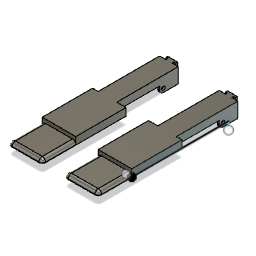
WhiteKeyCLRNew (Autodesk Fusion 360 design; units mm, degrees)
Autodesk Fusion 360 part; units mm, degrees
sketch "Sketch1" plane through (0, 0, 0) normal (0, 1, 0) x (1, 0, 0)
  line L0 (43.1546, -52.768) -> (20.2946, -52.768)
  line L1 (43.1546, -18.478) -> (43.1546, -52.768)
  line L2 (20.2946, -52.768) -> (20.2946, -50.8)
  line L3 (38.1, 23.432) -> (22.86, 23.432)
  line L4 (20.2946, -18.478) -> (20.2946, -52.768)
  line L5 (20.2946, -18.478) -> (22.86, -18.478)
  line L6 (22.86, -18.478) -> (22.86, 23.432)
  line L7 (38.1, 23.432) -> (38.1, -18.478)
  line L8 (38.1, -18.478) -> (43.1546, -18.478)
  dimension "d3" = 22.86
  dimension "d91" = 15.24
  dimension "d119" = 76.2
  dimension "d157" = 5.0546
  constraint horizontal L0
  constraint perpendicular L0 L2
  constraint perpendicular L1 L3
  constraint perpendicular L0 L4
  constraint perpendicular L4 L5
  constraint perpendicular L3 L6
  constraint perpendicular L3 L7
  constraint perpendicular L1 L8
  measures "d3" distance of L0.start L0.end
  measures "d91" distance of L3.end L3.start
  measures "d119" distance of L0 L3
  measures "d157" distance of L7.end L1.start
extrude "Extrude1" add sketch "Sketch1" along normal blind 5.08 makes body 1
sketch "Sketch18" plane through (0, 0, 0) normal (0, -1, 0) x (1, 0, 0)
  line L0 (22.86, -23.432) -> (38.1, -23.432)
  line L1 (38.1, -23.432) -> (38.1, 18.478)
  line L2 (38.1, 18.478) -> (43.1546, 18.478)
  line L3 (43.1546, 18.478) -> (43.1546, 52.768)
  line L4 (43.1546, 52.768) -> (20.2946, 52.768)
  line L5 (20.2946, 52.768) -> (20.2946, 18.478)
  line L6 (20.2946, 18.478) -> (22.86, 18.478)
  line L7 (22.86, 18.478) -> (22.86, -23.432)
  line L8 (35.56, -20.892) -> (35.56, 21.018)
  line L9 (35.56, 21.018) -> (40.6146, 21.018)
  line L10 (40.6146, 21.018) -> (40.6146, 50.228)
  line L11 (40.6146, 50.228) -> (22.8346, 50.228)
  line L12 (22.8346, 50.228) -> (22.8346, 21.018)
  line L13 (22.8346, 21.018) -> (25.4, 21.018)
  line L14 (35.56, -20.892) -> (25.4, -20.892)
  line L15 (25.4, -20.892) -> (25.4, 21.018)
  dimension "d130" = 2.54
  dimension "d131" = 2.54
  dimension "d132" = 2.54
  dimension "d133" = 2.54
  dimension "d134" = 2.54
  dimension "d135" = 2.54
  dimension "d136" = 2.54
  dimension "d137" = 2.54
  constraint perpendicular L0 L8
  constraint perpendicular L8 L9
  constraint perpendicular L9 L10
  constraint perpendicular L10 L11
  constraint perpendicular L11 L12
  constraint perpendicular L12 L13
  constraint perpendicular L8 L14
  constraint perpendicular L14 L15
  measures "d130" distance of L1 L8
  measures "d131" distance of L7 L15
  measures "d132" distance of L0 L14
  measures "d133" distance of L5 L12
  measures "d134" distance of L6 L13
  measures "d135" distance of L2 L9
  measures "d136" distance of L3 L10
  measures "d137" distance of L4 L11
extrude "Extrude20" cut sketch "Sketch18" against normal blind 3.81 contours L8 L9 L10 L11 L12 L13 L14 L15 bodies 1
sketch "Sketch19" plane through (0, 0, 0) normal (0, -1, 0) x (1, 0, 0)
  line L0 (40.6146, 21.018) -> (35.56, 21.018)
  line L1 (35.56, 21.018) -> (35.56, -20.892)
  line L2 (35.56, -20.892) -> (25.4, -20.892)
  line L3 (25.4, -20.892) -> (25.4, 21.018)
  line L4 (25.4, 21.018) -> (22.8346, 21.018)
  line L5 (22.8346, 21.018) -> (22.8346, 50.228)
  line L6 (22.8346, 50.228) -> (40.6146, 50.228)
  line L7 (40.6146, 50.228) -> (40.6146, 21.018)
  line L8 (22.86, -23.432) -> (38.1, -23.432)
  line L9 (38.1, -23.432) -> (38.1, 18.478)
  line L10 (38.1, 18.478) -> (43.1546, 18.478)
  line L11 (43.1546, 18.478) -> (43.1546, 52.768)
  line L12 (43.1546, 52.768) -> (20.2946, 52.768)
  line L13 (20.2946, 52.768) -> (20.2946, 18.478)
  line L14 (20.2946, 18.478) -> (22.86, 18.478)
  line L15 (22.86, 18.478) -> (22.86, -23.432)
  line L16 (35.56, -10.732) -> (38.1, -10.732)
  line L17 (38.1, -10.732) -> (38.1, -23.432)
  line L18 (38.1, -23.432) -> (35.56, -23.432)
  line L19 (35.56, -23.432) -> (35.56, -10.732)
  line L20 (22.86, -10.732) -> (26.162, -10.732)
  line L21 (26.162, -10.732) -> (26.162, -23.432)
  line L22 (26.162, -23.432) -> (22.86, -23.432)
  line L23 (22.86, -23.432) -> (22.86, -10.732)
  line L24 (25.4, -20.892) -> (35.56, -20.892)
  line L25 (35.56, -20.892) -> (35.56, -23.432)
  line L26 (35.56, -23.432) -> (25.4, -23.432)
  line L27 (25.4, -23.432) -> (25.4, -20.892)
  dimension "d149" = 12.7
  dimension "d150" = 12.7
  constraint horizontal L16
  constraint vertical L17
  constraint horizontal L18
  constraint vertical L19
  constraint coincident L8.end L9.start
  constraint coincident L1 L16.start
  constraint horizontal L20
  constraint vertical L21
  constraint horizontal L22
  constraint vertical L23
  constraint coincident L8 L21.end
  constraint coincident L15 L20.start
  constraint horizontal L24
  constraint vertical L25
  constraint horizontal L26
  constraint vertical L27
  constraint coincident L2.end L3.start
  measures "d149" distance of L16.start L18.end
  measures "d150" distance of L20.end L21.end
extrude "Extrude21" add sketch "Sketch19" along normal blind 5.08 contours L1 L8 L9 L16 L17 L18 L19 L25 | L3 L8 L15 L20 L22 L23 L27 bodies 1
fillet "Fillet7" radius 2.54 2 edges at (36.83, -5.08, -10.732) (24.13, -5.08, -10.732) on bodies 1
sketch "Sketch20" plane through (0, 0, 0) normal (0, -1, 0) x (1, 0, 0)
  line L0 (38.1, -10.732) -> (38.1, 18.478)
  line L1 (38.1, 18.478) -> (43.1546, 18.478)
  line L2 (43.1546, 18.478) -> (43.1546, 52.768)
  line L3 (43.1546, 52.768) -> (20.2946, 52.768)
  line L4 (20.2946, 52.768) -> (20.2946, 18.478)
  line L5 (20.2946, 18.478) -> (22.86, 18.478)
  line L6 (22.86, 18.478) -> (22.86, -10.732)
  line L7 (25.4, -10.732) -> (25.4, 21.018)
  line L8 (25.4, 21.018) -> (22.8346, 21.018)
  line L9 (22.8346, 21.018) -> (22.8346, 50.228)
  line L10 (22.8346, 50.228) -> (40.6146, 50.228)
  line L11 (40.6146, 50.228) -> (40.6146, 21.018)
  line L12 (40.6146, 21.018) -> (35.56, 21.018)
  line L13 (35.56, 21.018) -> (35.56, -10.732)
  line L14 (22.86, 18.478) -> (25.4, 18.478)
  line L15 (25.4, 18.478) -> (25.4, 12.3012)
  line L16 (25.4, 12.3012) -> (22.86, 12.3012)
  line L17 (22.86, 12.3012) -> (22.86, 18.478)
  line L18 (38.1, 18.478) -> (35.56, 18.478)
  line L19 (35.56, 18.478) -> (35.56, 12.3012)
  line L20 (35.56, 12.3012) -> (38.1, 12.3012)
  line L21 (38.1, 12.3012) -> (38.1, 18.478)
  line L22 (22.86, -10.732) -> (25.4, -10.732)
  line L23 (35.56, -10.732) -> (38.1, -10.732)
  constraint horizontal L14
  constraint vertical L15
  constraint horizontal L16
  constraint vertical L17
  constraint coincident L7 L15.end
  constraint coincident L5.end L6.start
  constraint horizontal L18
  constraint vertical L19
  constraint horizontal L20
  constraint vertical L21
  constraint coincident L13 L19.end
  constraint coincident L0.end L1.start
sketch "Sketch22" plane through (0, 0, -23.432) normal (0, 0, -1) x (-1, 0, 0)
  line L0 (-22.86, -5.08) -> (-22.86, 5.08)
  line L1 (-22.86, 5.08) -> (-38.1, 5.08)
  line L2 (-38.1, 5.08) -> (-38.1, -5.08)
  line L3 (-25.4, -5.08) -> (-22.86, -5.08)
  line L4 (-38.1, 5.08) -> (-22.86, 5.08)
  line L5 (-22.86, 5.08) -> (-22.86, 0)
  line L6 (-22.86, 0) -> (-38.1, 0)
  line L7 (-38.1, 0) -> (-38.1, 5.08)
  line L8 (-35.56, 0) -> (-25.4, 0)
  line L9 (-25.4, 0) -> (-25.4, -5.08)
  line L10 (-38.1, -5.08) -> (-35.56, -5.08)
  line L11 (-35.56, -5.08) -> (-35.56, 0)
  constraint horizontal L4
  constraint vertical L5
  constraint horizontal L6
  constraint vertical L7
  constraint midpoint L0 L5.end
  constraint coincident L1.end L2.start
extrude "Extrude24" add sketch "Sketch22" along normal blind 2.54 contours L0 L1 L2 L4 L5 L6 L7 L8 bodies 1
sketch "Sketch23" plane through (38.1, 0, 0) normal (1, 0, 0) x (0, 0, -1)
  arc A0 (10.732, -2.54) -> (13.272, -5.08) centre (13.272, -2.54) ccw
  line L0 (13.272, -5.08) -> (23.432, -5.08)
  line L1 (23.432, -5.08) -> (23.432, 0)
  line L2 (23.432, 0) -> (25.972, 0)
  line L3 (25.972, 0) -> (25.972, 5.08)
  line L4 (25.972, 5.08) -> (-18.478, 5.08)
  line L5 (-18.478, 5.08) -> (-18.478, 0)
  line L6 (-18.478, 0) -> (10.732, 0)
  line L7 (23.432, 0) -> (24.702, 0)
  line L8 (24.702, 0) -> (24.702, 3.81)
  line L9 (24.702, 3.81) -> (23.432, 3.81)
  line L10 (23.432, 3.81) -> (23.432, 0)
  line L11 (10.732, 0) -> (10.732, -2.54)
  dimension "d160" = 1.27
  constraint horizontal L7
  constraint vertical L8
  constraint horizontal L9
  constraint vertical L10
  constraint coincident L1.end L2.start
  measures "d160" distance of L1.end L7.end
extrude "Extrude25" cut sketch "Sketch23" against normal blind 1.27 contours L2 L7 L8 L9 L10 bodies 1
sketch "Sketch24" plane through (22.86, 0, 0) normal (-1, 0, 0) x (0, 0, 1)
  arc A0 (-13.272, -5.08) -> (-10.732, -2.54) centre (-13.272, -2.54) ccw
  line L0 (-10.732, 0) -> (18.478, 0)
  line L1 (18.478, 0) -> (18.478, 5.08)
  line L2 (18.478, 5.08) -> (-25.972, 5.08)
  line L3 (-25.972, 5.08) -> (-25.972, 0)
  line L4 (-25.972, 0) -> (-23.432, 0)
  line L5 (-23.432, 0) -> (-23.432, -5.08)
  line L6 (-23.432, -5.08) -> (-13.272, -5.08)
  line L7 (-23.432, 0) -> (-24.702, 0)
  line L8 (-24.702, 0) -> (-24.702, 3.81)
  line L9 (-24.702, 3.81) -> (-23.432, 3.81)
  line L10 (-23.432, 3.81) -> (-23.432, 0)
  line L11 (-10.732, -2.54) -> (-10.732, 0)
  dimension "d163" = 1.27
  constraint horizontal L7
  constraint vertical L8
  constraint horizontal L9
  constraint vertical L10
  constraint coincident L4.end L5.start
  measures "d163" distance of L4.end L7.end
extrude "Extrude26" cut sketch "Sketch24" against normal blind 1.27 contours L4 L7 L8 L9 L10 bodies 1
move_body "Move1" bodies 1 to x (1, 0, 0) y (0, 1, 0) z (0, 0, 1) at (-50.8, 0, 0)
sketch "Sketch25" plane through (0, 0, 52.768) normal (0, 0, 1) x (1, 0, 0)
  line L0 (-30.5054, 0) -> (-7.6454, 0)
  line L1 (-7.6454, 0) -> (-7.6454, 5.08)
  line L2 (-7.6454, 5.08) -> (-30.5054, 5.08)
  line L3 (-30.5054, 5.08) -> (-30.5054, 0)
  line L4 (-30.5054, 2.54) -> (-7.6454, 2.54)
  constraint midpoint L3 L4.start
  constraint midpoint L1 L4.end
extrude "Extrude27" add sketch "Sketch25" along normal blind 22.86 contours L0 L1 L3 L4 bodies 1
fillet "Fillet8" radius 2.286 5 edges at (-7.6454, 1.27, 75.628) (-7.6454, 2.54, 64.198) (-19.0754, 2.54, 75.628) (-30.5054, 2.54, 64.198) (-30.5054, 1.27, 75.628) on bodies 1
sketch "Sketch26" plane through (-12.7, 0, 0) normal (1, 0, 0) x (0, 0, -1)
  line L0 (23.432, -5.08) -> (23.432, 3.81)
  line L1 (25.972, 5.08) -> (-18.478, 5.08)
  line L2 (-18.478, 5.08) -> (-18.478, 0)
  line L3 (24.702, 0) -> (25.972, 0)
  line L4 (10.732, 0) -> (10.732, -2.54)
  arc A0 (10.732, -2.54) -> (13.272, -5.08) centre (13.272, -2.54) ccw
  line L5 (13.272, -5.08) -> (23.432, -5.08)
  circle A1 centre (13.272, -2.54) radius 1.27
  line L6 (24.702, 3.81) -> (24.702, 0)
  line L7 (25.972, 0) -> (25.972, 5.08)
  line L8 (23.432, 3.81) -> (24.702, 3.81)
  line L9 (-18.478, 0) -> (10.732, 0)
  dimension "d174" = 2.54
  constraint concentric A0 A1
  measures "d174" diameter of A1
extrude "Extrude28" cut sketch "Sketch26" against normal blind 25.4 contours A1 bodies 1
mirror "Mirror4" about plane through (0, 0, 0) normal (1, 0, 0) of bodies 1 makes body 2
extrude "Extrude29" cut 1 faces at (26.67, 1.27, -23.8553) along direction (-1, 0, 0) blind 1.27 on bodies 2 bodies 2
extrude "Extrude30" cut 1 faces at (27.94, -1.2069, -20.4639) along direction (-1, 0, 0) blind 1.27 on bodies 2 bodies 2
extrude "Extrude31" cut 1 faces at (13.97, 1.27, -23.8553) along direction (1, 0, 0) blind 1.27 on bodies 2 bodies 2
extrude "Extrude32" cut 1 faces at (12.7, -1.2069, -20.4639) along direction (1, 0, 0) blind 1.27 on bodies 2 bodies 2
extrude "Extrude33" cut 1 faces at (-13.97, 1.27, -23.8553) along direction (-1, 0, 0) blind 1.27 on bodies 1 bodies 1
extrude "Extrude34" cut 1 faces at (-12.7, -1.2069, -20.4639) along direction (-1, 0, 0) blind 1.27 on bodies 1 bodies 1
extrude "Extrude35" cut 1 faces at (-26.67, 1.27, -23.8553) along direction (1, 0, 0) blind 1.27 on bodies 1 bodies 1
extrude "Extrude36" cut 1 faces at (-27.94, -1.2069, -20.4639) along direction (1, 0, 0) blind 1.27 on bodies 1 bodies 1
extrude "Extrude37" cut 1 faces at (26.2467, 3.81, -24.2787) along direction (0, 1, 0) blind 3.302 on bodies 2 bodies 2
extrude "Extrude38" cut 1 faces at (14.3933, 3.81, -24.2787) along direction (0, 1, 0) blind 3.556 on bodies 2 bodies 2
extrude "Extrude39" cut 1 faces at (-26.2467, 3.81, -24.2787) along direction (0, 1, 0) blind 1.27 on bodies 1 bodies 1
extrude "Extrude40" cut 1 faces at (-14.3933, 3.81, -24.2787) along direction (0, 1, 0) blind 2.794 on bodies 1 bodies 1
sketch "Sketch28" plane through (0, 5.08, 0) normal (0, 1, 0) x (-1, 0, 0)
  line L0 (-15.24, -23.432) -> (-13.97, -23.432)
  line L1 (-13.97, -23.432) -> (-13.97, 18.478)
  line L2 (-13.97, 18.478) -> (-7.6454, 18.478)
  line L3 (-7.6454, 18.478) -> (-7.6454, 52.768)
  line L4 (-7.6454, 52.768) -> (-30.5054, 52.768)
  line L5 (-30.5054, 52.768) -> (-30.5054, 18.478)
  line L6 (-30.5054, 18.478) -> (-26.67, 18.478)
  line L7 (-26.67, 18.478) -> (-26.67, -23.432)
  line L8 (-26.67, -23.432) -> (-25.4, -23.432)
  line L9 (-25.4, -23.432) -> (-25.4, -24.702)
  line L10 (-25.4, -24.702) -> (-26.67, -24.702)
  line L11 (-26.67, -24.702) -> (-26.67, -25.972)
  line L12 (-26.67, -25.972) -> (-13.97, -25.972)
  line L13 (-13.97, -25.972) -> (-13.97, -24.702)
  line L14 (-13.97, -24.702) -> (-15.24, -24.702)
  line L15 (-15.24, -24.702) -> (-15.24, -23.432)
  line L16 (-20.32, -25.972) -> (-20.32, -23.432)
  line L17 (-20.32, -25.972) -> (-16.9545, -25.972)
  line L18 (-20.32, -25.972) -> (-23.6855, -25.972)
  line L19 (-23.6855, -25.972) -> (-23.6855, -24.702)
  line L20 (-23.6855, -24.702) -> (-22.4155, -24.702)
  line L21 (-22.4155, -24.702) -> (-22.4155, -23.432)
  line L22 (-22.4155, -23.432) -> (-20.32, -23.432)
  line L23 (-16.9545, -25.972) -> (-16.9545, -24.702)
  line L24 (-16.9545, -24.702) -> (-18.2245, -24.702)
  line L25 (-18.2245, -24.702) -> (-18.2245, -23.432)
  line L26 (-18.2245, -23.432) -> (-20.32, -23.432)
  line L27 (-15.24, -23.432) -> (-18.2245, -23.432)
  line L28 (-22.4155, -23.432) -> (-25.4, -23.432)
  line L29 (-13.97, -25.972) -> (-13.97, -24.702)
  line L30 (-15.24, -24.702) -> (-15.24, -23.432)
  line L31 (-13.97, -25.972) -> (-16.9545, -25.972)
  line L32 (-23.6855, -25.972) -> (-26.67, -25.972)
  line L33 (-26.67, -24.702) -> (-25.4, -24.702)
  line L34 (-25.4, -23.7416) -> (-25.4, -24.702)
  line L35 (-26.67, -25.972) -> (-26.67, -24.702)
  line L36 (-23.6855, -25.972) -> (-26.67, -25.972)
  dimension "d204" = 3.3655
  dimension "d205" = 3.3655
  dimension "d206" = 1.27
  dimension "d207" = 1.27
  dimension "d208" = 1.27
  dimension "d209" = 1.27
  dimension "d210" = 1.27
  dimension "d211" = 1.27
  constraint midpoint L12 L16.start
  constraint perpendicular L12 L16
  constraint perpendicular L16 L17
  constraint perpendicular L16 L18
  constraint perpendicular L12 L19
  constraint perpendicular L19 L20
  constraint perpendicular L20 L21
  constraint perpendicular L16 L22
  constraint perpendicular L12 L23
  constraint perpendicular L23 L24
  constraint perpendicular L24 L25
  constraint coincident L0.start L15.end
  constraint coincident L8.end L9.start
  constraint coincident L12.end L13.start
  constraint coincident L13.end L14.start
  constraint coincident L14.end L15.start
  constraint coincident L11.end L12.start
  constraint coincident L10.end L11.start
  constraint coincident L9.end L10.start
  constraint coincident L9 L34.start
  constraint perpendicular L10 L34
  measures "d204" distance of L16.start L17.end
  measures "d205" distance of L16.start L18.end
  measures "d206" distance of L18.end L19.end
  measures "d207" distance of L19.end L20.end
  measures "d208" distance of L20.end L21.end
  measures "d209" distance of L17.end L23.end
  measures "d210" distance of L23.end L24.end
  measures "d211" distance of L24.end L25.end
extrude "Extrude41" cut sketch "Sketch28" against normal blind 5.08 contours L12 L13 L14 L15 L23 L24 L25 L27 L29 L30 L31 | L9 L10 L11 L12 L19 L20 L21 L28 L32 L33 L34 L35 L36 bodies 2
sketch "Sketch29" plane through (0, 5.08, 0) normal (0, 1, 0) x (-1, 0, 0)
  line L0 (15.24, -24.702) -> (13.97, -24.702)
  line L1 (13.97, -24.702) -> (13.97, -25.972)
  line L2 (13.97, -25.972) -> (26.67, -25.972)
  line L3 (26.67, -25.972) -> (26.67, -24.702)
  line L4 (26.67, -24.702) -> (25.4, -24.702)
  line L5 (25.4, -24.702) -> (25.4, -23.432)
  line L6 (25.4, -23.432) -> (26.67, -23.432)
  line L7 (26.67, -23.432) -> (26.67, 18.478)
  line L8 (26.67, 18.478) -> (30.5054, 18.478)
  line L9 (30.5054, 18.478) -> (30.5054, 52.768)
  line L10 (30.5054, 52.768) -> (7.6454, 52.768)
  line L11 (7.6454, 52.768) -> (7.6454, 18.478)
  line L12 (7.6454, 18.478) -> (13.97, 18.478)
  line L13 (13.97, 18.478) -> (13.97, -23.432)
  line L14 (13.97, -23.432) -> (15.24, -23.432)
  line L15 (15.24, -23.432) -> (15.24, -24.702)
  line L16 (20.32, -25.972) -> (20.32, -23.432)
  line L17 (20.32, -25.972) -> (23.6855, -25.972)
  line L18 (20.32, -25.972) -> (16.9418, -25.972)
  line L19 (16.9418, -25.972) -> (16.9418, -24.702)
  line L20 (16.9418, -24.702) -> (18.2118, -24.702)
  line L21 (18.2118, -24.702) -> (18.2118, -23.432)
  line L22 (23.6855, -25.972) -> (23.6855, -24.702)
  line L23 (23.6855, -24.702) -> (22.4155, -24.702)
  line L24 (22.4155, -24.702) -> (22.4155, -23.432)
  line L25 (22.4155, -23.432) -> (20.32, -23.432)
  line L26 (20.32, -23.432) -> (18.2118, -23.432)
  line L27 (22.4155, -23.432) -> (25.4, -23.432)
  line L28 (25.4, -24.702) -> (25.4, -23.432)
  line L29 (25.4, -24.702) -> (26.67, -24.702)
  line L30 (26.67, -25.972) -> (26.67, -24.702)
  line L31 (26.67, -25.972) -> (23.6855, -25.972)
  line L32 (18.2118, -23.432) -> (15.24, -23.432)
  line L33 (15.24, -24.702) -> (15.24, -23.432)
  line L34 (15.24, -24.702) -> (13.97, -24.702)
  line L35 (13.97, -25.972) -> (13.97, -24.702)
  line L36 (13.97, -25.972) -> (16.9418, -25.972)
  dimension "d215" = 3.3655
  dimension "d216" = 3.3782
  dimension "d217" = 1.27
  dimension "d218" = 1.27
  dimension "d219" = 1.27
  dimension "d220" = 1.27
  dimension "d221" = 1.27
  constraint midpoint L2 L16.start
  constraint perpendicular L2 L16
  constraint perpendicular L16 L17
  constraint perpendicular L16 L18
  constraint perpendicular L2 L19
  constraint perpendicular L19 L20
  constraint perpendicular L20 L21
  constraint perpendicular L17 L22
  constraint perpendicular L22 L23
  constraint perpendicular L23 L24
  constraint perpendicular L21 L26
  constraint coincident L5.end L6.start
  constraint coincident L4.end L5.start
  constraint coincident L3.end L4.start
  constraint coincident L2.end L3.start
  constraint coincident L14.end L15.start
  constraint perpendicular L15 L32
  constraint coincident L0.start L15.end
  constraint coincident L0.end L1.start
  constraint coincident L1.end L2.start
  measures "d215" distance of L16.start L17.end
  measures "d216" distance of L16.start L18.end
  measures "d217" distance of L18.end L19.end
  measures "d218" distance of L19.end L20.end
  measures "d219" distance of L17.end L22.end
  measures "d220" distance of L22.end L23.end
  measures "d221" distance of L23.end L24.end
extrude "Extrude42" cut sketch "Sketch29" against normal blind 5.08 contours L0 L1 L2 L15 L19 L20 L21 L32 L33 L34 L35 L36 | L2 L3 L4 L5 L22 L23 L24 L27 L28 L29 L30 L31 bodies 1
sketch "Sketch30" plane through (26.67, 0, 0) normal (1, 0, 0) x (0, 0, -1)
  line L0 (23.432, -5.08) -> (23.432, 5.08)
  line L1 (23.432, 5.08) -> (-18.478, 5.08)
  line L2 (-18.478, 5.08) -> (-18.478, 0)
  line L3 (-18.478, 0) -> (10.732, 0)
  line L4 (10.732, 0) -> (10.732, -2.54)
  arc A0 (10.732, -2.54) -> (13.272, -5.08) centre (13.272, -2.54) ccw
  line L5 (13.272, -5.08) -> (23.432, -5.08)
  circle A1 centre (13.272, -2.54) radius 1.27
  line L6 (-52.761, 0.2532) -> (-52.761, 0)
  constraint vertical L6
sketch "Sketch31" plane through (0, 3.81, 0) normal (0, -1, 0) x (1, 0, 0)
  line L0 (15.24, 21.018) -> (15.24, -20.892)
  line L1 (15.24, -20.892) -> (25.4, -20.892)
  line L2 (25.4, -20.892) -> (25.4, 21.018)
  line L3 (25.4, 21.018) -> (27.9654, 21.018)
  line L4 (27.9654, 21.018) -> (27.9654, 50.228)
  line L5 (27.9654, 50.228) -> (10.1854, 50.228)
  line L6 (10.1854, 50.228) -> (10.1854, 21.018)
  line L7 (10.1854, 21.018) -> (15.24, 21.018)
  line L8 (19.0754, 38.798) -> (15.9004, 38.798)
  line L9 (19.0754, 38.798) -> (22.2504, 38.798)
  line L10 (22.2504, 38.798) -> (22.2504, 35.623)
  line L11 (22.2504, 35.623) -> (22.2504, 32.448)
  line L12 (15.9004, 38.798) -> (15.9004, 35.623)
  line L13 (15.9004, 35.623) -> (15.9004, 32.448)
  line L14 (15.9004, 32.448) -> (22.2504, 32.448)
  line L15 (10.1854, 35.623) -> (15.9004, 35.623)
  line L16 (22.2504, 35.623) -> (27.9654, 35.623)
  line L17 (19.0754, 50.228) -> (19.0754, 38.798)
  line L18 (19.0754, 32.448) -> (19.0754, 20.32)
  dimension "d229" = 3.175
  dimension "d230" = 3.175
  dimension "d231" = 3.175
  dimension "d232" = 3.175
  dimension "d233" = 3.175
  constraint midpoint L5 L17.start
  constraint perpendicular L5 L17
  constraint midpoint L6 L15.start
  constraint midpoint L4 L16.end
  constraint coincident L10.end L15
  constraint perpendicular L10 L15
  constraint perpendicular L11 L15
  constraint perpendicular L8 L12
  constraint perpendicular L13 L15
  constraint perpendicular L11 L14
  constraint collinear L15 L16
  constraint coincident L14 L18.start
  constraint collinear L17 L18
  measures "d229" distance of L8.start L8.end
  measures "d230" distance of L8.start L9.end
  measures "d231" distance of L10.end L11.end
  measures "d232" distance of L8.end L12.end
  measures "d233" distance of L12.end L13.end
sketch "Sketch32" plane through (0, 3.81, 0) normal (0, -1, 0) x (1, 0, 0)
  line L0 (-15.24, -20.892) -> (-15.24, 21.018)
  line L1 (-15.24, 21.018) -> (-10.1854, 21.018)
  line L2 (-10.1854, 21.018) -> (-10.1854, 50.228)
  line L3 (-10.1854, 50.228) -> (-27.9654, 50.228)
  line L4 (-27.9654, 50.228) -> (-27.9654, 21.018)
  line L5 (-27.9654, 21.018) -> (-25.4, 21.018)
  line L6 (-25.4, 21.018) -> (-25.4, -20.892)
  line L7 (-25.4, -20.892) -> (-15.24, -20.892)
  line L8 (-19.0754, 38.798) -> (-15.9004, 38.798)
  line L9 (-15.9004, 38.798) -> (-15.9004, 35.623)
  line L10 (-19.0754, 38.798) -> (-22.2504, 38.798)
  line L11 (-22.2504, 38.798) -> (-22.2504, 32.448)
  line L12 (-22.2504, 32.448) -> (-15.9004, 32.448)
  line L13 (-15.9004, 35.623) -> (-15.9004, 32.448)
  line L14 (-27.9654, 35.623) -> (-22.2504, 35.623)
  line L15 (-15.9004, 35.623) -> (-10.1854, 35.623)
  line L16 (-19.0754, 50.228) -> (-19.0754, 38.798)
  line L17 (-19.0754, 32.448) -> (-19.0754, 20.32)
  dimension "d235" = 3.175
  dimension "d236" = 3.175
  dimension "d237" = 3.175
  dimension "d238" = 6.35
  dimension "d239" = 6.35
  constraint midpoint L3 L16.start
  constraint perpendicular L3 L16
  constraint midpoint L4 L14.start
  constraint midpoint L2 L15.end
  constraint perpendicular L8 L9
  constraint perpendicular L10 L16
  constraint perpendicular L10 L11
  constraint perpendicular L11 L12
  constraint coincident L11 L14.end
  constraint collinear L14 L15
  constraint collinear L16 L17
  constraint coincident L12 L17.start
  measures "d235" distance of L8.start L8.end
  measures "d236" distance of L8.end L9.end
  measures "d237" distance of L8.start L10.end
  measures "d238" distance of L10.end L11.end
  measures "d239" distance of L11.end L12.end
extrude "Extrude43" add sketch "Sketch32" sketch "Sketch31" along normal blind 8.89 contours L8 L9 L10 L11 L12 L13 of sketch 2 contours L8 L9 L10 L11 L12 L13 L14 bodies 1 2
sketch "Sketch33" plane through (22.2504, 0, 0) normal (1, 0, 0) x (0, 0, -1)
  line L0 (-32.448, 3.81) -> (-38.798, 3.81)
  line L1 (-38.798, 3.81) -> (-38.798, -5.08)
  line L2 (-38.798, -5.08) -> (-32.448, -5.08)
  line L3 (-32.448, -5.08) -> (-32.448, 3.81)
  line L4 (13.208, -2.54) -> (13.208, -5.08)
  line L5 (13.208, -2.54) -> (13.208, 0)
  line L6 (-32.448, 0.0071) -> (-32.448, -2.5089)
  line L7 (-38.798, 0.0984) -> (-38.798, -1.9096)
  line L8 (-38.798, -1.9096) -> (-32.448, -2.5089)
  line L9 (-38.798, -1.9096) -> (-38.798, -5.08)
  line L10 (-32.448, -5.08) -> (-38.798, -5.08)
  line L11 (-32.448, -2.5089) -> (-32.448, -5.08)
  dimension "d242" = 2.516
  dimension "d243" = 2.008
  constraint perpendicular L2 L4
  constraint parallel L4 L5
  constraint coincident L3 L6.start
  constraint perpendicular L0 L6
  constraint coincident L1 L7.start
  constraint parallel L1 L7
  constraint coincident L1.end L2.start
  constraint perpendicular L2 L9
  constraint coincident L2.end L3.start
  measures "d242" distance of L6.start L6.end
  measures "d243" distance of L7.start L7.end
extrude "Extrude44" cut sketch "Sketch33" against normal blind 53.34 contours L1 L2 L3 L8 L9 L10 L11 bodies 1 2
sketch "Sketch34" plane through (30.5054, 0, 0) normal (1, 0, 0) x (0, 0, -1)
  line L0 (-73.342, 0.254) -> (-73.342, 0)
  line L1 (-73.342, 0) -> (-18.478, 0)
  line L2 (-18.478, 0) -> (-18.478, 5.08)
  line L3 (-18.478, 5.08) -> (-52.768, 5.08)
  line L4 (-52.768, 5.08) -> (-52.768, 0.254)
  line L5 (-52.768, 0.254) -> (-73.342, 0.254)
  line L6 (-52.768, 0.254) -> (13.2548, 0.254)
  line L7 (13.2548, 0.254) -> (13.2548, -5.08)
  constraint coincident L4.end L5.start
  constraint perpendicular L4 L6
  constraint perpendicular L6 L7
equation "d204 = ( 0.265 / 2 ) * 1 in"
equation "d205 = ( 0.265 / 2 ) * 1 in"
equation "d215 = ( 0.265 / 2 ) * 1 in"
equation "d242 = 0.04 in + 1.5 mm"
equation "d243 = 0.02 in + 1.5 mm"
